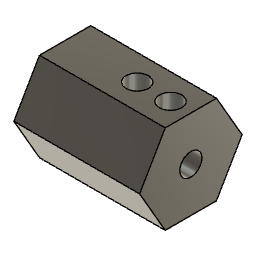
Buggy (Autodesk Fusion 360 archive; units mm, degrees)
design "HexAdapter"
Autodesk Fusion 360 part; units mm, degrees
(part 1 of 3)
sketch "Sketch1" plane through (0, 0, 0) normal (1, 0, 0) x (0, 1, 0)
  line L0 (3.4641, -6) -> (6.9282, 0)
  line L1 (6.9282, 0) -> (3.4641, 6)
  line L2 (3.4641, 6) -> (-3.4641, 6)
  line L3 (-3.4641, 6) -> (-6.9282, 0)
  line L4 (-6.9282, 0) -> (-3.4641, -6)
  line L5 (-3.4641, -6) -> (3.4641, -6)
  dimension "d1" = 6
  measures "d1" distance of origin L5
extrude "Extrude1" add sketch "Sketch1" along normal blind 17
sketch "Sketch2" plane through (0, 0, 0) normal (-1, 0, 0) x (0, -1, 0)
  line L0 (-3.4641, -6) -> (3.4641, -6)
  line L1 (3.4641, -6) -> (6.9282, 0)
  line L2 (6.9282, 0) -> (3.4641, 6)
  line L3 (3.4641, 6) -> (-3.4641, 6)
  line L4 (-3.4641, 6) -> (-6.9282, 0)
  line L5 (-6.9282, 0) -> (-3.4641, -6)
  circle A0 centre (0, 0) radius 1.5
  dimension "d4" = 3
  constraint coincident A0.centre origin
  measures "d4" diameter of A0
extrude "Extrude2" cut sketch "Sketch2" against normal blind 31 contours A0
sketch "Sketch3" plane through (0, 0, 6) normal (0, 0, 1) x (-1, 0, 0)
  line L0 (0, -3.4641) -> (0, 3.4641)
  line L1 (0, 3.4641) -> (-17, 3.4641)
  line L2 (-17, 3.4641) -> (-17, -3.4641)
  line L3 (-17, -3.4641) -> (0, -3.4641)
  line L4 (-17, 0) -> (-14.25, 0)
  circle A0 centre (-14.25, 0) radius 1.5
  line L5 (-14.25, 0) -> (-9.75, 0)
  circle A1 centre (-9.75, 0) radius 1.5
  dimension "d7" = 2.75
  dimension "d8" = 3
  dimension "d9" = 4.5
  dimension "d10" = 3
  constraint midpoint L2 L4.start
  constraint perpendicular L2 L4
  constraint coincident L4.end A0.centre
  constraint parallel L4 L5
  constraint coincident L5.end A1.centre
  measures "d7" distance of L4.start L4.end
  measures "d8" diameter of A0
  measures "d9" distance of L4.end L5.end
  measures "d10" diameter of A1
extrude "Extrude3" cut sketch "Sketch3" against normal blind 6 contours L4 A0 L5 | L4 A0 L5 | A1

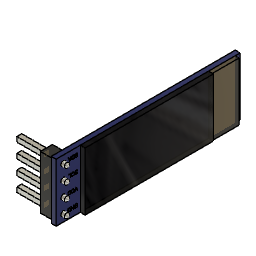
design "OLED mini display"
Autodesk Fusion 360 part; units mm, degrees
sketch "Sketch1" plane through (0, 0, 0) normal (1, 0, 0) x (0, 1, 0)
  line L0 (19, 6) -> (-19, 6)
  line L1 (-19, 6) -> (-19, -6)
  line L2 (-19, -6) -> (19, -6)
  line L3 (19, -6) -> (19, 6)
  line L4 (19, 6) -> (-19, -6) construction
  line L5 (-19, 6) -> (19, -6) construction
  dimension "d1" = 38
  dimension "d2" = 12
  constraint horizontal L0
  constraint perpendicular L0 L1
  constraint parallel L0 L2
  constraint parallel L1 L3
  constraint coincident L4 origin
  constraint coincident L5 origin
  measures "d1" distance of L1.end L2.end
  measures "d2" distance of L0.end L1.end
extrude "Extrude1" add sketch "Sketch1" along normal blind 1 makes body 1
sketch "Sketch2" plane through (1, 0, 0) normal (1, 0, 0) x (0, 1, 0)
  line L0 (19, -6) -> (19, 6)
  line L1 (19, 6) -> (-19, 6)
  line L2 (-19, 6) -> (-19, -6)
  line L3 (-19, -6) -> (19, -6)
  line L4 (-19, 6) -> (-14, 6)
  line L5 (-14, 6) -> (-14, -6)
  line L6 (-14, -6) -> (-19, -6)
  line L7 (-19, -6) -> (-19, 6)
  line L8 (-19, 6) -> (-18, 6)
  line L9 (-18, 6) -> (-18, -6)
  line L10 (-18, 4.5) -> (-18, -4.5)
  circle A0 centre (-17.5, 4.5) radius 0.5
  circle A1 centre (-17.5, 1.5) radius 0.5
  circle A2 centre (-17.5, -1.5) radius 0.5
  circle A3 centre (-17.5, -4.5) radius 0.5
  line L11 (19, 6) -> (18, 6)
  line L12 (18, 6) -> (18, -6)
  line L13 (18, -6) -> (19, -6)
  line L14 (19, -6) -> (19, 6)
  line L15 (18, -6) -> (12.5, -6)
  line L16 (12.5, -6) -> (12.5, 6)
  line L17 (18, 6) -> (12.5, 6)
  line L18 (-14, 6) -> (12.5, 6)
  line L19 (12.5, -6) -> (-14, -6)
  dimension "d5" = 5
  dimension "d6" = 1
  dimension "d7" = 9
  dimension "d8" = 1
  dimension "d11" = 0
  dimension "d12" = -9
  dimension "d13" = 1
  dimension "d14" = 5.5
  constraint coincident L1.end L2.start
  constraint perpendicular L2 L4
  constraint coincident L3 L5.end
  constraint perpendicular L3 L5
  constraint coincident L2.end L3.start
  constraint perpendicular L7 L8
  constraint coincident L6 L9.end
  constraint perpendicular L3 L10
  constraint midpoint L9 L10
  constraint coincident L10.start A0
  constraint coincident L0.end L1.start
  constraint perpendicular L0 L11
  constraint coincident L3 L12.end
  constraint perpendicular L3 L12
  constraint coincident L0.start L3.end
  constraint perpendicular L12 L15
  constraint coincident L1 L16.end
  constraint perpendicular L1 L16
  measures "d5" distance of L1.end L4.end
  measures "d6" distance of L1.end L8.end
  measures "d7" distance of L10.start L10.end
  measures "d8" diameter of A0
  measures "d13" distance of L0.end L11.end
  measures "d14" distance of L12.end L15.end
extrude "Extrude2" add sketch "Sketch2" along normal blind 1 separate body contours L1 L3 L5 L16 L18 L19 makes body 2
extrude "Extrude3" add sketch "Sketch2" along normal blind 0.8 separate body contours L1 L3 L12 L15 L16 L17 makes body 3
extrude "Extrude4" add sketch "Sketch2" along normal blind 1.2 contours A0 | A1 | A2 | A3 bodies 1
chamfer "Chamfer1" distance 0.5 angle 45 4 faces at (2.2, -17.7632, 4.6455) (2.2, -17.7632, 1.6455) (2.2, -17.7632, -1.3545) (2.2, -17.3907, -4.6662) on bodies 1
sketch "Sketch3" plane through (0, 0, 0) normal (-1, 0, 0) x (0, -1, 0)
  line L0 (-19, 6) -> (-19, -6)
  line L1 (-19, -6) -> (19, -6)
  line L2 (19, -6) -> (19, 6)
  line L3 (19, 6) -> (-19, 6)
  line L4 (17, -5) -> (18, -5)
  line L5 (18, -5) -> (18, -4)
  line L6 (18, -4) -> (17, -4)
  line L7 (17, -4) -> (17, -5)
  line L8 (17, -5) -> (18, -4) construction
  line L9 (18, -5) -> (17, -4) construction
  line L10 (17, -2) -> (18, -2)
  line L11 (18, -2) -> (18, -1)
  line L12 (18, -1) -> (17, -1)
  line L13 (17, -1) -> (17, -2)
  line L14 (17, -2) -> (18, -1) construction
  line L15 (18, -2) -> (17, -1) construction
  line L16 (17, 1) -> (18, 1)
  line L17 (18, 1) -> (18, 2)
  line L18 (18, 2) -> (17, 2)
  line L19 (17, 2) -> (17, 1)
  line L20 (17, 1) -> (18, 2) construction
  line L21 (18, 1) -> (17, 2) construction
  line L22 (17, 4) -> (18, 4)
  line L23 (18, 4) -> (18, 5)
  line L24 (18, 5) -> (17, 5)
  line L25 (17, 5) -> (17, 4)
  line L26 (17, 4) -> (18, 5) construction
  line L27 (18, 4) -> (17, 5) construction
  point P0 (17.5, -4.5)
  point P1 (17.5, -1.5)
  point P2 (17.5, 1.5)
  point P3 (17.5, 4.5)
  constraint horizontal L4
  constraint perpendicular L4 L5
  constraint parallel L4 L6
  constraint parallel L5 L7
  constraint coincident L8 P0
  constraint coincident L9 P0
  constraint horizontal L10
  constraint perpendicular L10 L11
  constraint parallel L10 L12
  constraint parallel L11 L13
  constraint coincident L14 P1
  constraint coincident L15 P1
  constraint horizontal L16
  constraint perpendicular L16 L17
  constraint parallel L16 L18
  constraint parallel L17 L19
  constraint coincident L20 P2
  constraint coincident L21 P2
  constraint horizontal L22
  constraint perpendicular L22 L23
  constraint parallel L22 L24
  constraint parallel L23 L25
  constraint coincident L26 P3
  constraint coincident L27 P3
extrude "Extrude5" add sketch "Sketch3" along normal blind 8.5 contours L4 L5 L6 L7 | L10 L11 L12 L13 | L16 L17 L18 L19 | L22 L23 L24 L25 bodies 1
chamfer "Chamfer2" distance 0.4 angle 45 4 faces at (-8.5, -17.3333, -4.3333) (-8.5, -17.3333, -1.3333) (-8.5, -17.3333, 1.6667) (-8.5, -17.3333, 4.6667) on bodies 1
sketch "Sketch4" plane through (0, 0, 0) normal (-1, 0, 0) x (0, -1, 0)
  line L0 (17, 5) -> (18, 5)
  line L1 (18, 5) -> (18, 4)
  line L2 (18, 4) -> (17, 4)
  line L3 (17, 4) -> (17, 5)
  line L4 (17, -4) -> (18, -4)
  line L5 (18, -4) -> (18, -5)
  line L6 (18, -5) -> (17, -5)
  line L7 (17, -5) -> (17, -4)
  line L8 (17, 2) -> (18, 2)
  line L9 (18, 2) -> (18, 1)
  line L10 (18, 1) -> (17, 1)
  line L11 (17, 1) -> (17, 2)
  line L12 (17, -1) -> (18, -1)
  line L13 (18, -1) -> (18, -2)
  line L14 (18, -2) -> (17, -2)
  line L15 (17, -2) -> (17, -1)
  line L16 (-19, 6) -> (-19, -6)
  line L17 (-19, -6) -> (19, -6)
  line L18 (19, -6) -> (19, 6)
  line L19 (19, 6) -> (-19, 6)
  line L20 (19, -5.5) -> (19, 5.5)
  line L21 (19, -5.5) -> (18.75, -5.5)
  line L22 (18.75, -5.5) -> (16.25, -5.5)
  line L23 (18.75, -5.5) -> (18.75, 5.5)
  line L24 (18.75, 5.5) -> (16.25, 5.5)
  line L25 (16.25, 5.5) -> (16.25, -5.5)
  dimension "d25" = 11
  dimension "d27" = 11
  constraint vertical L20
  constraint midpoint L18 L20
  constraint perpendicular L20 L21
  constraint perpendicular L21 L23
  constraint perpendicular L23 L24
  constraint perpendicular L22 L25
  measures "d25" distance of L20.start L20.end
  measures "d27" distance of L21.end L23.end
extrude "Extrude6" add sketch "Sketch4" along normal blind 2.5 contours L22 L23 L24 L25 bodies 1
sketch "Sketch5" plane through (1, 0, 0) normal (1, 0, 0) x (0, 1, 0)
  circle A0 centre (-17.5, -4.5) radius 0.5
  circle A1 centre (-17.5, 4.5) radius 0.5
  circle A2 centre (-17.5, -1.5) radius 0.5
  circle A3 centre (-17.5, 1.5) radius 0.5
  line L0 (19, -6) -> (19, 6)
  line L1 (19, 6) -> (-19, 6)
  line L2 (-19, 6) -> (-19, -6)
  line L3 (-19, -6) -> (19, -6)
  line L4 (-14.5293, -4) -> (-16.5, -4) construction
  line L5 (-16.5, -4) -> (-16.5, -4.767) construction
  line L6 (-16.5, -4.767) -> (-14.5293, -4.767) construction
  line L7 (-14.5293, -4.767) -> (-14.5293, -4) construction
  line L8 (-14.5293, -1) -> (-16.5, -1) construction
  line L9 (-16.5, -1) -> (-16.5, -1.767) construction
  line L10 (-16.5, -1.767) -> (-14.5293, -1.767) construction
  line L11 (-14.5293, -1.767) -> (-14.5293, -1) construction
  line L12 (-14.5293, 2) -> (-16.5, 2) construction
  line L13 (-16.5, 2) -> (-16.5, 1.233) construction
  line L14 (-16.5, 1.233) -> (-14.5293, 1.233) construction
  line L15 (-14.5293, 1.233) -> (-14.5293, 2) construction
  line L16 (-14.5293, 5) -> (-16.5, 5) construction
  line L17 (-16.5, 5) -> (-16.5, 4.233) construction
  line L18 (-16.5, 4.233) -> (-14.5293, 4.233) construction
  line L19 (-14.5293, 4.233) -> (-14.5293, 5) construction
  dimension "d30" = 0.7
  dimension "d31" = 0.7
  dimension "d32" = 0.7
  dimension "d33" = 0.7
  text T0 "GND" font "Arial" height 0.7 align left top in box 1.9707 x 0.767 at (-14.5293, -4) x (-1, 0) y (0, -1) spacing 1 kerned
  text T1 "VCC" font "Arial" height 0.7 align left top in box 1.9707 x 0.767 at (-14.5293, -1) x (-1, 0) y (0, -1) spacing 1 kerned
  text T2 "SCL" font "Arial" height 0.7 align left top in box 1.9707 x 0.767 at (-14.5293, 2) x (-1, 0) y (0, -1) spacing 1 kerned
  text T3 "SDA" font "Arial" height 0.7 align left top in box 1.9707 x 0.767 at (-14.5293, 5) x (-1, 0) y (0, -1) spacing 1 kerned
extrude "Extrude7" cut sketch "Sketch5" against normal blind 0.5 text T0 T1 T2 T3 bodies 1

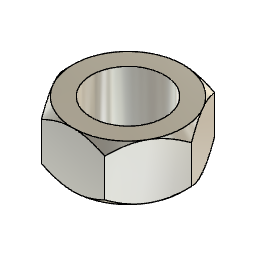
design "2mm Nut"
Autodesk Fusion 360 part; units mm, degrees
sketch "Sketch1" plane through (0, 0, 0) normal (0, 0, 1) x (1, 0, 0)
  circle A0 centre (0, 0) radius 1
  line L0 (-0.866, 1.5) -> (-1.7321, 0)
  line L1 (-1.7321, 0) -> (-0.866, -1.5)
  line L2 (-0.866, -1.5) -> (0.866, -1.5)
  line L3 (0.866, -1.5) -> (1.7321, 0)
  line L4 (1.7321, 0) -> (0.866, 1.5)
  line L5 (0.866, 1.5) -> (-0.866, 1.5)
  dimension "d1" = 2
  constraint coincident A0.centre origin
  measures "d1" diameter of A0
extrude "Extrude1" add sketch "Sketch1" along normal blind 1.5
sketch "Sketch2" plane through (0, 0, 1.5) normal (0, 0, 1) x (-1, 0, 0)
  circle A0 centre (0, 0) radius 1
  line L0 (-0.866, -1.5) -> (0.866, -1.5)
  line L1 (0.866, -1.5) -> (1.7321, 0)
  line L2 (1.7321, 0) -> (0.866, 1.5)
  line L3 (0.866, 1.5) -> (-0.866, 1.5)
  line L4 (-0.866, 1.5) -> (-1.7321, 0)
  line L5 (-1.7321, 0) -> (-0.866, -1.5)
  circle A1 centre (0, 0) radius 1.5
  constraint coincident A0.centre A1.centre
  constraint tangent L0 A1
extrude "Extrude2" cut sketch "Sketch2" against normal blind 3 draft 45 contours A1 keep common part
sketch "Sketch3" plane through (0, 0, 0) normal (0, 0, -1) x (1, 0, 0)
  circle A0 centre (0, 0) radius 1
  line L0 (-0.866, -1.5) -> (0.866, -1.5)
  line L1 (0.866, -1.5) -> (1.7321, 0)
  line L2 (1.7321, 0) -> (0.866, 1.5)
  line L3 (0.866, 1.5) -> (-0.866, 1.5)
  line L4 (-0.866, 1.5) -> (-1.7321, 0)
  line L5 (-1.7321, 0) -> (-0.866, -1.5)
  circle A1 centre (0, 0) radius 1.5
  constraint concentric A0 A1
  constraint tangent L3 A1
extrude "Extrude3" cut sketch "Sketch3" against normal blind 4.4 draft 45 contours A1 keep common part

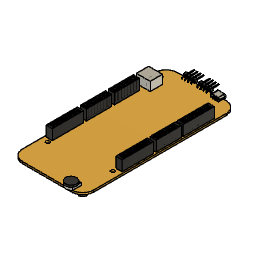
design "S32k144"
Autodesk Fusion 360 part; units mm, degrees
sketch "Sketch1" plane through (0, 0, 0) normal (0, 0, 1) x (1, 0, 0)
  line L0 (0, 0) -> (20, 0)
  line L1 (0, 0) -> (-20, 0)
  line L2 (0, 0) -> (0, 126)
  line L3 (-29, 9) -> (-29, 117)
  line L4 (-20, 126) -> (20, 126)
  line L5 (29, 117) -> (29, 9)
  arc A0 (-20, 126) -> (-29, 117) centre (-20, 117) ccw
  arc A1 (29, 117) -> (20, 126) centre (20, 117) ccw
  arc A2 (20, 0) -> (29, 9) centre (20, 9) ccw
  arc A3 (-29, 9) -> (-20, 0) centre (-20, 9) ccw
  line L6 (-29, 117) -> (-29, 116)
  line L7 (-29, 116) -> (-23.5, 116) construction
  line L8 (-23.5, 116) -> (-23.5, 125.2916) construction
  circle A4 centre (-23.5, 116) radius 1.5
  line L9 (-23.5, 116) -> (-23.5, 24) construction
  circle A5 centre (-23.5, 24) radius 1.5
  line L10 (29, 0) -> (29, 30) construction
  line L11 (29, 30) -> (23.5, 30) construction
  circle A6 centre (23.5, 30) radius 1.5
  line L12 (23.5, 30) -> (23.5, 110) construction
  circle A7 centre (23.5, 110) radius 1.5
  line L13 (29, 108.5) -> (27.7, 108.5) construction
  line L14 (27.7, 108.5) -> (22.7, 108.5)
  line L15 (22.7, 108.5) -> (22.7, 83)
  line L16 (27.7, 108.5) -> (27.7, 83)
  line L17 (22.7, 83) -> (27.7, 83)
  line L18 (25.2, 83) -> (25.2, 81.7) construction
  line L19 (22.7, 81.7) -> (27.7, 81.7)
  line L20 (27.7, 81.7) -> (27.7, 61.2)
  line L21 (22.7, 81.7) -> (22.7, 61.2)
  line L22 (22.7, 61.2) -> (27.7, 61.2)
  line L23 (25.2, 61.2) -> (25.2, 58.9) construction
  line L24 (22.7, 58.9) -> (27.7, 58.9)
  line L25 (27.7, 58.9) -> (27.7, 33.4)
  line L26 (22.7, 58.9) -> (22.7, 33.4)
  line L27 (22.7, 33.4) -> (27.7, 33.4)
  line L28 (-23.5, 116) -> (-23.5, 98) construction
  line L29 (-29, 98) -> (-27.7, 98) construction
  line L30 (-27.7, 98) -> (-22.7, 98)
  line L31 (-27.7, 98) -> (-27.7, 77.5)
  line L32 (-27.7, 77.5) -> (-22.7, 77.5)
  line L33 (-22.7, 98) -> (-22.7, 77.5)
  line L34 (-25.2, 77.5) -> (-25.2, 75.2) construction
  line L35 (-27.7, 75.2) -> (-22.7, 75.2)
  line L36 (-22.7, 75.2) -> (-22.7, 54.7)
  line L37 (-27.7, 75.2) -> (-27.7, 54.7)
  line L38 (-27.7, 54.7) -> (-22.7, 54.7)
  line L39 (-25.2, 54.7) -> (-25.2, 52.4) construction
  line L40 (-27.7, 52.4) -> (-22.7, 52.4)
  line L41 (-27.7, 52.4) -> (-27.7, 26.9)
  line L42 (-22.7, 52.4) -> (-22.7, 26.9)
  line L43 (-27.7, 26.9) -> (-22.7, 26.9)
  line L44 (-25.2, 98) -> (-25.2, 101.5) construction
  line L45 (-29, 101.5) -> (-29, 111.5)
  line L46 (-29, 111.5) -> (-17.5, 111.5)
  line L47 (-17.5, 111.5) -> (-17.5, 101.5)
  line L48 (-17.5, 101.5) -> (-29, 101.5)
  line L49 (-29, 111.5) -> (-28.75, 111.5)
  line L50 (-28.75, 111.5) -> (-28.75, 101.5)
  point P0 (29, 0)
  point P1 (-29, 0)
  point P2 (-29, 126)
  point P3 (29, 126)
  dimension "d1" = 29
  dimension "d2" = 29
  dimension "d3" = 126
  dimension "d4" = 126
  dimension "d5" = 58
  dimension "d6" = 9
  dimension "d7" = 9
  dimension "d8" = 9
  dimension "d9" = 9
  dimension "d13" = 1
  dimension "d15" = 5.5
  dimension "d16" = 9.2916
  dimension "d17" = 3
  dimension "d18" = 92
  dimension "d19" = 3
  dimension "d20" = 30
  dimension "d21" = 5.5
  dimension "d22" = 3
  dimension "d23" = 80
  dimension "d24" = 3
  dimension "d26" = 1.3
  dimension "d27" = 5
  dimension "d29" = 25.5
  dimension "d30" = 1.3
  dimension "d31" = 5
  dimension "d32" = 20.5
  dimension "d34" = 2.3
  dimension "d35" = 5
  dimension "d36" = 25.5
  dimension "d38" = 18
  dimension "d39" = 1.3
  dimension "d40" = 5
  dimension "d41" = 20.5
  dimension "d42" = 5
  dimension "d43" = 2.3
  dimension "d44" = 5
  dimension "d46" = 20.5
  dimension "d47" = 2.3
  dimension "d48" = 5
  dimension "d49" = 25.5
  dimension "d51" = 3.5
  dimension "d52" = 10
  dimension "d53" = 11.5
  dimension "d54" = 10
  dimension "d61" = 0.25
  constraint coincident L0.start L1.start
  constraint horizontal L0
  constraint parallel L0 L1
  constraint perpendicular L0 L2
  constraint perpendicular L1 L3
  constraint perpendicular L2 L4
  constraint coincident P2 L3
  constraint coincident P2 L4
  constraint tangent L3 A0
  constraint tangent L4 A0
  constraint coincident P3 L4
  constraint coincident P3 L5
  constraint tangent L4 A1
  constraint tangent L5 A1
  constraint coincident P0 L0
  constraint coincident P0 L5
  constraint tangent L0 A2
  constraint tangent L5 A2
  constraint coincident P1 L1
  constraint coincident P1 L3
  constraint tangent L1 A3
  constraint tangent L3 A3
  constraint parallel L3 L6
  constraint coincident A0 L8.end
  constraint perpendicular L7 L8
  constraint coincident L7.end L8.start
  constraint perpendicular L7 L9
  constraint coincident L9.end A5.centre
  constraint coincident P0 L10.start
  constraint parallel L5 L10
  constraint perpendicular L5 L11
  constraint coincident L11.end A6.centre
  constraint perpendicular L11 L12
  constraint coincident L12.end A7.centre
  constraint coincident L5 L13.start
  constraint perpendicular L5 L13
  constraint parallel L13 L14
  constraint perpendicular L14 L15
  constraint perpendicular L14 L16
  constraint midpoint L17 L18.start
  constraint perpendicular L17 L18
  constraint perpendicular L18 L19
  constraint perpendicular L19 L20
  constraint perpendicular L19 L21
  constraint tangent A7 L14
  constraint midpoint L22 L23.start
  constraint perpendicular L22 L23
  constraint perpendicular L12 L24
  constraint perpendicular L24 L25
  constraint perpendicular L24 L26
  constraint perpendicular L7 L28
  constraint coincident L3 L29.start
  constraint perpendicular L3 L29
  constraint parallel L29 L30
  constraint perpendicular L30 L31
  constraint perpendicular L31 L32
  constraint midpoint L32 L34.start
  constraint perpendicular L32 L34
  constraint perpendicular L9 L35
  constraint perpendicular L35 L36
  constraint perpendicular L35 L37
  constraint midpoint L38 L39.start
  constraint perpendicular L38 L39
  constraint perpendicular L39 L40
  constraint perpendicular L40 L41
  constraint perpendicular L40 L42
  constraint midpoint L30 L44.start
  constraint perpendicular L30 L44
  constraint coincident L3 L45.start
  constraint parallel L3 L45
  constraint perpendicular L45 L46
  constraint perpendicular L46 L47
  constraint perpendicular L45 L49
  constraint coincident L48 L50.end
  constraint perpendicular L48 L50
  measures "d1" distance of L0.start P0
  measures "d2" distance of L0.start P1
  measures "d3" distance of L0.start L2.end
  measures "d4" distance of P1 P2
  measures "d5" distance of P2 P3
  measures "d6" radius of A0
  measures "d7" radius of A1
  measures "d8" radius of A2
  measures "d9" radius of A3
  measures "d13" distance of L3.end L6.end
  measures "d15" distance of L6.end L7.end
  measures "d16" distance of L7.end L8.end
  measures "d17" diameter of A4
  measures "d18" distance of L7.end L9.end
  measures "d19" diameter of A5
  measures "d20" distance of P0 L10.end
  measures "d21" distance of L10.end L11.end
  measures "d22" diameter of A6
  measures "d23" distance of L11.end L12.end
  measures "d24" diameter of A7
  measures "d26" distance of L13.start L13.end
  measures "d27" distance of L13.end L14.end
  measures "d29" distance of L13.end L16.end
  measures "d30" distance of L18.start L18.end
  measures "d31" distance of L19.start L19.end
  measures "d32" distance of L19.end L20.end
  measures "d34" distance of L23.start L23.end
  measures "d35" distance of L24.start L24.end
  measures "d36" distance of L24.end L25.end
  measures "d38" distance of L7.end L28.end
  measures "d39" distance of L29.start L29.end
  measures "d40" distance of L29.end L30.end
  measures "d41" distance of L29.end L31.end
  measures "d42" distance of L31.end L32.end
  measures "d43" distance of L34.start L34.end
  measures "d44" distance of L35.start L35.end
  measures "d46" distance of L35.start L37.end
  measures "d47" distance of L39.start L39.end
  measures "d48" distance of L40.start L40.end
  measures "d49" distance of L40.start L41.end
  measures "d51" distance of L44.start L44.end
  measures "d52" distance of L45.start L45.end
  measures "d53" distance of L45.end L46.end
  measures "d54" distance of L46.end L47.end
  measures "d61" distance of L45.end L49.end
extrude "Extrude1" add sketch "Sketch1" along normal blind 1.5 contours L0 L2 L4 L5 A1 A2 | L1 L2 L3 L4 A0 A3 L6 L46 L47 L48 L49 | L3 L45 L46 L48 L49 L50 | L46 L47 L48 L50 | A4 | A5 | A6 | A7 | L14 L15 L16 L17 | L19 L20 L21 L22 | L24 L25 L26 L27 | L30 L31 L32 L33 | L35 L36 L37 L38 | L40 L41 L42 L43 makes body 1
extrude "Extrude2" cut sketch "Sketch1" along normal blind 33 contours A4 | A5 | A6 | A7 bodies 1
extrude "Extrude3" add sketch "Sketch1" along normal blind 10 contours L14 L15 L16 L17 | L19 L20 L21 L22 | L24 L25 L26 L27 | L30 L31 L32 L33 | L35 L36 L37 L38 | L40 L41 L42 L43 bodies 1
extrude "Extrude4" add sketch "Sketch1" along normal blind 8.7 contours L46 L47 L48 L50 bodies 1
sketch "Sketch2" plane through (-28.75, 0, 0) normal (-1, 0, 0) x (0, -1, 0)
  line L0 (-111.5, 1.5) -> (-101.5, 1.5)
  line L1 (-101.5, 1.5) -> (-101.5, 8.7)
  line L2 (-101.5, 8.7) -> (-111.5, 8.7)
  line L3 (-111.5, 8.7) -> (-111.5, 1.5)
  circle A0 centre (-105, 5) radius 3
  dimension "d64" = 6
  measures "d64" diameter of A0
extrude "Extrude5" cut sketch "Sketch2" against normal blind 8 contours A0 bodies 1
sketch "Sketch3" plane through (-20.75, 0, 0) normal (-1, 0, 0) x (0, -1, 0)
  circle A0 centre (-105, 5) radius 3
  circle A1 centre (-105, 5) radius 1
  dimension "d67" = 2
  constraint concentric A0 A1
  measures "d67" diameter of A1
extrude "Extrude6" add sketch "Sketch3" along normal blind 7 contours A1 bodies 1
fillet "Fillet1" radius 1 1 faces at (-27.75, 105.0787, 4.4037) on bodies 1
sketch "Sketch4" plane through (0, 0, 10) normal (0, 0, 1) x (-1, 0, 0)
  line L0 (27.7, -98) -> (27.7, -77.5)
  line L1 (27.7, -77.5) -> (22.7, -77.5)
  line L2 (22.7, -77.5) -> (22.7, -98)
  line L3 (22.7, -98) -> (27.7, -98)
  line L4 (27, -97) -> (25.5, -97)
  line L5 (25.5, -97) -> (25.5, -95.5)
  line L6 (25.5, -95.5) -> (27, -95.5)
  line L7 (27, -95.5) -> (27, -97)
  line L8 (24.7, -97) -> (23.2, -97)
  line L9 (24.7, -95.5) -> (24.7, -97)
  line L10 (23.2, -95.5) -> (24.7, -95.5)
  line L11 (23.2, -97) -> (23.2, -95.5)
  line L12 (27, -94.5714) -> (25.5, -94.5714)
  line L13 (27, -93.0714) -> (27, -94.5714)
  line L14 (25.5, -93.0714) -> (27, -93.0714)
  line L15 (25.5, -94.5714) -> (25.5, -93.0714)
  line L16 (24.7, -94.5714) -> (23.2, -94.5714)
  line L17 (24.7, -93.0714) -> (24.7, -94.5714)
  line L18 (23.2, -93.0714) -> (24.7, -93.0714)
  line L19 (23.2, -94.5714) -> (23.2, -93.0714)
  line L20 (27, -92.1429) -> (25.5, -92.1429)
  line L21 (27, -90.6429) -> (27, -92.1429)
  line L22 (25.5, -90.6429) -> (27, -90.6429)
  line L23 (25.5, -92.1429) -> (25.5, -90.6429)
  line L24 (24.7, -92.1429) -> (23.2, -92.1429)
  line L25 (24.7, -90.6429) -> (24.7, -92.1429)
  line L26 (23.2, -90.6429) -> (24.7, -90.6429)
  line L27 (23.2, -92.1429) -> (23.2, -90.6429)
  line L28 (27, -89.7143) -> (25.5, -89.7143)
  line L29 (27, -88.2143) -> (27, -89.7143)
  line L30 (25.5, -88.2143) -> (27, -88.2143)
  line L31 (25.5, -89.7143) -> (25.5, -88.2143)
  line L32 (24.7, -89.7143) -> (23.2, -89.7143)
  line L33 (24.7, -88.2143) -> (24.7, -89.7143)
  line L34 (23.2, -88.2143) -> (24.7, -88.2143)
  line L35 (23.2, -89.7143) -> (23.2, -88.2143)
  line L36 (27, -87.2857) -> (25.5, -87.2857)
  line L37 (27, -85.7857) -> (27, -87.2857)
  line L38 (25.5, -85.7857) -> (27, -85.7857)
  line L39 (25.5, -87.2857) -> (25.5, -85.7857)
  line L40 (24.7, -87.2857) -> (23.2, -87.2857)
  line L41 (24.7, -85.7857) -> (24.7, -87.2857)
  line L42 (23.2, -85.7857) -> (24.7, -85.7857)
  line L43 (23.2, -87.2857) -> (23.2, -85.7857)
  line L44 (27, -84.8571) -> (25.5, -84.8571)
  line L45 (27, -83.3571) -> (27, -84.8571)
  line L46 (25.5, -83.3571) -> (27, -83.3571)
  line L47 (25.5, -84.8571) -> (25.5, -83.3571)
  line L48 (24.7, -84.8571) -> (23.2, -84.8571)
  line L49 (24.7, -83.3571) -> (24.7, -84.8571)
  line L50 (23.2, -83.3571) -> (24.7, -83.3571)
  line L51 (23.2, -84.8571) -> (23.2, -83.3571)
  line L52 (27, -82.4286) -> (25.5, -82.4286)
  line L53 (27, -80.9286) -> (27, -82.4286)
  line L54 (25.5, -80.9286) -> (27, -80.9286)
  line L55 (25.5, -82.4286) -> (25.5, -80.9286)
  line L56 (24.7, -82.4286) -> (23.2, -82.4286)
  line L57 (24.7, -80.9286) -> (24.7, -82.4286)
  line L58 (23.2, -80.9286) -> (24.7, -80.9286)
  line L59 (23.2, -82.4286) -> (23.2, -80.9286)
  line L60 (27, -80) -> (25.5, -80)
  line L61 (27, -78.5) -> (27, -80)
  line L62 (25.5, -78.5) -> (27, -78.5)
  line L63 (25.5, -80) -> (25.5, -78.5)
  line L64 (24.7, -80) -> (23.2, -80)
  line L65 (24.7, -78.5) -> (24.7, -80)
  line L66 (23.2, -78.5) -> (24.7, -78.5)
  line L67 (23.2, -80) -> (23.2, -78.5)
  line L68 (27, -74) -> (25.5, -74)
  line L69 (27, -72.5) -> (27, -74)
  line L70 (25.5, -72.5) -> (27, -72.5)
  line L71 (25.5, -74) -> (25.5, -72.5)
  line L72 (27, -51) -> (25.5, -51)
  line L73 (27, -49.5) -> (27, -51)
  line L74 (25.5, -49.5) -> (27, -49.5)
  line L75 (25.5, -51) -> (25.5, -49.5)
  line L76 (-23.5, -56) -> (-23.5, -57.5)
  line L77 (-25, -57.5) -> (-25, -56)
  line L78 (-25, -56) -> (-23.5, -56)
  line L79 (-23.5, -57.5) -> (-25, -57.5)
  line L80 (-23.5, -78.5) -> (-23.5, -80)
  line L81 (-25, -80) -> (-25, -78.5)
  line L82 (-25, -78.5) -> (-23.5, -78.5)
  line L83 (-23.5, -80) -> (-25, -80)
  line L84 (-25, -107) -> (-25, -105.5)
  line L85 (-23.5, -105.5) -> (-23.5, -107)
  line L86 (-23.5, -107) -> (-25, -107)
  line L87 (-25, -105.5) -> (-23.5, -105.5)
  line L88 (24.7, -74) -> (23.2, -74)
  line L89 (24.7, -72.5) -> (24.7, -74)
  line L90 (23.2, -74) -> (23.2, -72.5)
  line L91 (23.2, -72.5) -> (24.7, -72.5)
  line L92 (27, -71.5714) -> (25.5, -71.5714)
  line L93 (27, -70.0714) -> (27, -71.5714)
  line L94 (25.5, -71.5714) -> (25.5, -70.0714)
  line L95 (25.5, -70.0714) -> (27, -70.0714)
  line L96 (24.7, -71.5714) -> (23.2, -71.5714)
  line L97 (24.7, -70.0714) -> (24.7, -71.5714)
  line L98 (23.2, -71.5714) -> (23.2, -70.0714)
  line L99 (23.2, -70.0714) -> (24.7, -70.0714)
  line L100 (27, -69.1429) -> (25.5, -69.1429)
  line L101 (27, -67.6429) -> (27, -69.1429)
  line L102 (25.5, -69.1429) -> (25.5, -67.6429)
  line L103 (25.5, -67.6429) -> (27, -67.6429)
  line L104 (24.7, -69.1429) -> (23.2, -69.1429)
  line L105 (24.7, -67.6429) -> (24.7, -69.1429)
  line L106 (23.2, -69.1429) -> (23.2, -67.6429)
  line L107 (23.2, -67.6429) -> (24.7, -67.6429)
  line L108 (27, -66.7143) -> (25.5, -66.7143)
  line L109 (27, -65.2143) -> (27, -66.7143)
  line L110 (25.5, -66.7143) -> (25.5, -65.2143)
  line L111 (25.5, -65.2143) -> (27, -65.2143)
  line L112 (24.7, -66.7143) -> (23.2, -66.7143)
  line L113 (24.7, -65.2143) -> (24.7, -66.7143)
  line L114 (23.2, -66.7143) -> (23.2, -65.2143)
  line L115 (23.2, -65.2143) -> (24.7, -65.2143)
  line L116 (27, -64.2857) -> (25.5, -64.2857)
  line L117 (27, -62.7857) -> (27, -64.2857)
  line L118 (25.5, -64.2857) -> (25.5, -62.7857)
  line L119 (25.5, -62.7857) -> (27, -62.7857)
  line L120 (24.7, -64.2857) -> (23.2, -64.2857)
  line L121 (24.7, -62.7857) -> (24.7, -64.2857)
  line L122 (23.2, -64.2857) -> (23.2, -62.7857)
  line L123 (23.2, -62.7857) -> (24.7, -62.7857)
  line L124 (27, -61.8571) -> (25.5, -61.8571)
  line L125 (27, -60.3571) -> (27, -61.8571)
  line L126 (25.5, -61.8571) -> (25.5, -60.3571)
  line L127 (25.5, -60.3571) -> (27, -60.3571)
  line L128 (24.7, -61.8571) -> (23.2, -61.8571)
  line L129 (24.7, -60.3571) -> (24.7, -61.8571)
  line L130 (23.2, -61.8571) -> (23.2, -60.3571)
  line L131 (23.2, -60.3571) -> (24.7, -60.3571)
  line L132 (27, -59.4286) -> (25.5, -59.4286)
  line L133 (27, -57.9286) -> (27, -59.4286)
  line L134 (25.5, -59.4286) -> (25.5, -57.9286)
  line L135 (25.5, -57.9286) -> (27, -57.9286)
  line L136 (24.7, -59.4286) -> (23.2, -59.4286)
  line L137 (24.7, -57.9286) -> (24.7, -59.4286)
  line L138 (23.2, -59.4286) -> (23.2, -57.9286)
  line L139 (23.2, -57.9286) -> (24.7, -57.9286)
  line L140 (27, -57) -> (25.5, -57)
  line L141 (27, -55.5) -> (27, -57)
  line L142 (25.5, -57) -> (25.5, -55.5)
  line L143 (25.5, -55.5) -> (27, -55.5)
  line L144 (24.7, -57) -> (23.2, -57)
  line L145 (24.7, -55.5) -> (24.7, -57)
  line L146 (23.2, -57) -> (23.2, -55.5)
  line L147 (23.2, -55.5) -> (24.7, -55.5)
  line L148 (25, -51) -> (23.5, -51)
  line L149 (25, -49.5) -> (25, -51)
  line L150 (23.5, -49.5) -> (25, -49.5)
  line L151 (23.5, -51) -> (23.5, -49.5)
  line L152 (27, -48.6667) -> (25.5, -48.6667)
  line L153 (27, -47.1667) -> (27, -48.6667)
  line L154 (25.5, -47.1667) -> (27, -47.1667)
  line L155 (25.5, -48.6667) -> (25.5, -47.1667)
  line L156 (25, -48.6667) -> (23.5, -48.6667)
  line L157 (25, -47.1667) -> (25, -48.6667)
  line L158 (23.5, -47.1667) -> (25, -47.1667)
  line L159 (23.5, -48.6667) -> (23.5, -47.1667)
  line L160 (27, -46.3333) -> (25.5, -46.3333)
  line L161 (27, -44.8333) -> (27, -46.3333)
  line L162 (25.5, -44.8333) -> (27, -44.8333)
  line L163 (25.5, -46.3333) -> (25.5, -44.8333)
  line L164 (25, -46.3333) -> (23.5, -46.3333)
  line L165 (25, -44.8333) -> (25, -46.3333)
  line L166 (23.5, -44.8333) -> (25, -44.8333)
  line L167 (23.5, -46.3333) -> (23.5, -44.8333)
  line L168 (27, -44) -> (25.5, -44)
  line L169 (27, -42.5) -> (27, -44)
  line L170 (25.5, -42.5) -> (27, -42.5)
  line L171 (25.5, -44) -> (25.5, -42.5)
  line L172 (25, -44) -> (23.5, -44)
  line L173 (25, -42.5) -> (25, -44)
  line L174 (23.5, -42.5) -> (25, -42.5)
  line L175 (23.5, -44) -> (23.5, -42.5)
  line L176 (27, -41.6667) -> (25.5, -41.6667)
  line L177 (27, -40.1667) -> (27, -41.6667)
  line L178 (25.5, -40.1667) -> (27, -40.1667)
  line L179 (25.5, -41.6667) -> (25.5, -40.1667)
  line L180 (25, -41.6667) -> (23.5, -41.6667)
  line L181 (25, -40.1667) -> (25, -41.6667)
  line L182 (23.5, -40.1667) -> (25, -40.1667)
  line L183 (23.5, -41.6667) -> (23.5, -40.1667)
  line L184 (27, -39.3333) -> (25.5, -39.3333)
  line L185 (27, -37.8333) -> (27, -39.3333)
  line L186 (25.5, -37.8333) -> (27, -37.8333)
  line L187 (25.5, -39.3333) -> (25.5, -37.8333)
  line L188 (25, -39.3333) -> (23.5, -39.3333)
  line L189 (25, -37.8333) -> (25, -39.3333)
  line L190 (23.5, -37.8333) -> (25, -37.8333)
  line L191 (23.5, -39.3333) -> (23.5, -37.8333)
  line L192 (27, -37) -> (25.5, -37)
  line L193 (27, -35.5) -> (27, -37)
  line L194 (25.5, -35.5) -> (27, -35.5)
  line L195 (25.5, -37) -> (25.5, -35.5)
  line L196 (25, -37) -> (23.5, -37)
  line L197 (25, -35.5) -> (25, -37)
  line L198 (23.5, -35.5) -> (25, -35.5)
  line L199 (23.5, -37) -> (23.5, -35.5)
  line L200 (27, -34.6667) -> (25.5, -34.6667)
  line L201 (27, -33.1667) -> (27, -34.6667)
  line L202 (25.5, -33.1667) -> (27, -33.1667)
  line L203 (25.5, -34.6667) -> (25.5, -33.1667)
  line L204 (25, -34.6667) -> (23.5, -34.6667)
  line L205 (25, -33.1667) -> (25, -34.6667)
  line L206 (23.5, -33.1667) -> (25, -33.1667)
  line L207 (23.5, -34.6667) -> (23.5, -33.1667)
  line L208 (27, -32.3333) -> (25.5, -32.3333)
  line L209 (27, -30.8333) -> (27, -32.3333)
  line L210 (25.5, -30.8333) -> (27, -30.8333)
  line L211 (25.5, -32.3333) -> (25.5, -30.8333)
  line L212 (25, -32.3333) -> (23.5, -32.3333)
  line L213 (25, -30.8333) -> (25, -32.3333)
  line L214 (23.5, -30.8333) -> (25, -30.8333)
  line L215 (23.5, -32.3333) -> (23.5, -30.8333)
  line L216 (27, -30) -> (25.5, -30)
  line L217 (27, -28.5) -> (27, -30)
  line L218 (25.5, -28.5) -> (27, -28.5)
  line L219 (25.5, -30) -> (25.5, -28.5)
  line L220 (25, -30) -> (23.5, -30)
  line L221 (25, -28.5) -> (25, -30)
  line L222 (23.5, -28.5) -> (25, -28.5)
  line L223 (23.5, -30) -> (23.5, -28.5)
  line L224 (-27, -107) -> (-27, -105.5)
  line L225 (-25.5, -105.5) -> (-25.5, -107)
  line L226 (-27, -105.5) -> (-25.5, -105.5)
  line L227 (-25.5, -107) -> (-27, -107)
  line L228 (-25, -104.6667) -> (-25, -103.1667)
  line L229 (-23.5, -103.1667) -> (-23.5, -104.6667)
  line L230 (-25, -103.1667) -> (-23.5, -103.1667)
  line L231 (-23.5, -104.6667) -> (-25, -104.6667)
  line L232 (-27, -104.6667) -> (-27, -103.1667)
  line L233 (-25.5, -103.1667) -> (-25.5, -104.6667)
  line L234 (-27, -103.1667) -> (-25.5, -103.1667)
  line L235 (-25.5, -104.6667) -> (-27, -104.6667)
  line L236 (-25, -102.3333) -> (-25, -100.8333)
  line L237 (-23.5, -100.8333) -> (-23.5, -102.3333)
  line L238 (-25, -100.8333) -> (-23.5, -100.8333)
  line L239 (-23.5, -102.3333) -> (-25, -102.3333)
  line L240 (-27, -102.3333) -> (-27, -100.8333)
  line L241 (-25.5, -100.8333) -> (-25.5, -102.3333)
  line L242 (-27, -100.8333) -> (-25.5, -100.8333)
  line L243 (-25.5, -102.3333) -> (-27, -102.3333)
  line L244 (-25, -100) -> (-25, -98.5)
  line L245 (-23.5, -98.5) -> (-23.5, -100)
  line L246 (-25, -98.5) -> (-23.5, -98.5)
  line L247 (-23.5, -100) -> (-25, -100)
  line L248 (-27, -100) -> (-27, -98.5)
  line L249 (-25.5, -98.5) -> (-25.5, -100)
  line L250 (-27, -98.5) -> (-25.5, -98.5)
  line L251 (-25.5, -100) -> (-27, -100)
  line L252 (-25, -97.6667) -> (-25, -96.1667)
  line L253 (-23.5, -96.1667) -> (-23.5, -97.6667)
  line L254 (-25, -96.1667) -> (-23.5, -96.1667)
  line L255 (-23.5, -97.6667) -> (-25, -97.6667)
  line L256 (-27, -97.6667) -> (-27, -96.1667)
  line L257 (-25.5, -96.1667) -> (-25.5, -97.6667)
  line L258 (-27, -96.1667) -> (-25.5, -96.1667)
  line L259 (-25.5, -97.6667) -> (-27, -97.6667)
  line L260 (-25, -95.3333) -> (-25, -93.8333)
  line L261 (-23.5, -93.8333) -> (-23.5, -95.3333)
  line L262 (-25, -93.8333) -> (-23.5, -93.8333)
  line L263 (-23.5, -95.3333) -> (-25, -95.3333)
  line L264 (-27, -95.3333) -> (-27, -93.8333)
  line L265 (-25.5, -93.8333) -> (-25.5, -95.3333)
  line L266 (-27, -93.8333) -> (-25.5, -93.8333)
  line L267 (-25.5, -95.3333) -> (-27, -95.3333)
  line L268 (-25, -93) -> (-25, -91.5)
  line L269 (-23.5, -91.5) -> (-23.5, -93)
  line L270 (-25, -91.5) -> (-23.5, -91.5)
  line L271 (-23.5, -93) -> (-25, -93)
  line L272 (-27, -93) -> (-27, -91.5)
  line L273 (-25.5, -91.5) -> (-25.5, -93)
  line L274 (-27, -91.5) -> (-25.5, -91.5)
  line L275 (-25.5, -93) -> (-27, -93)
  line L276 (-25, -90.6667) -> (-25, -89.1667)
  line L277 (-23.5, -89.1667) -> (-23.5, -90.6667)
  line L278 (-25, -89.1667) -> (-23.5, -89.1667)
  line L279 (-23.5, -90.6667) -> (-25, -90.6667)
  line L280 (-27, -90.6667) -> (-27, -89.1667)
  line L281 (-25.5, -89.1667) -> (-25.5, -90.6667)
  line L282 (-27, -89.1667) -> (-25.5, -89.1667)
  line L283 (-25.5, -90.6667) -> (-27, -90.6667)
  line L284 (-25, -88.3333) -> (-25, -86.8333)
  line L285 (-23.5, -86.8333) -> (-23.5, -88.3333)
  line L286 (-25, -86.8333) -> (-23.5, -86.8333)
  line L287 (-23.5, -88.3333) -> (-25, -88.3333)
  line L288 (-27, -88.3333) -> (-27, -86.8333)
  line L289 (-25.5, -86.8333) -> (-25.5, -88.3333)
  line L290 (-27, -86.8333) -> (-25.5, -86.8333)
  line L291 (-25.5, -88.3333) -> (-27, -88.3333)
  line L292 (-25, -86) -> (-25, -84.5)
  line L293 (-23.5, -84.5) -> (-23.5, -86)
  line L294 (-25, -84.5) -> (-23.5, -84.5)
  line L295 (-23.5, -86) -> (-25, -86)
  line L296 (-27, -86) -> (-27, -84.5)
  line L297 (-25.5, -84.5) -> (-25.5, -86)
  line L298 (-27, -84.5) -> (-25.5, -84.5)
  line L299 (-25.5, -86) -> (-27, -86)
  line L300 (-27, -78.5) -> (-25.5, -78.5)
  line L301 (-27, -80) -> (-27, -78.5)
  line L302 (-25.5, -78.5) -> (-25.5, -80)
  line L303 (-25.5, -80) -> (-27, -80)
  line L304 (-25, -76.2143) -> (-23.5, -76.2143)
  line L305 (-25, -77.7143) -> (-25, -76.2143)
  line L306 (-23.5, -76.2143) -> (-23.5, -77.7143)
  line L307 (-23.5, -77.7143) -> (-25, -77.7143)
  line L308 (-27, -76.2143) -> (-25.5, -76.2143)
  line L309 (-27, -77.7143) -> (-27, -76.2143)
  line L310 (-25.5, -76.2143) -> (-25.5, -77.7143)
  line L311 (-25.5, -77.7143) -> (-27, -77.7143)
  line L312 (-25, -73.9286) -> (-23.5, -73.9286)
  line L313 (-25, -75.4286) -> (-25, -73.9286)
  line L314 (-23.5, -73.9286) -> (-23.5, -75.4286)
  line L315 (-23.5, -75.4286) -> (-25, -75.4286)
  line L316 (-27, -73.9286) -> (-25.5, -73.9286)
  line L317 (-27, -75.4286) -> (-27, -73.9286)
  line L318 (-25.5, -73.9286) -> (-25.5, -75.4286)
  line L319 (-25.5, -75.4286) -> (-27, -75.4286)
  line L320 (-25, -71.6429) -> (-23.5, -71.6429)
  line L321 (-25, -73.1429) -> (-25, -71.6429)
  line L322 (-23.5, -71.6429) -> (-23.5, -73.1429)
  line L323 (-23.5, -73.1429) -> (-25, -73.1429)
  line L324 (-27, -71.6429) -> (-25.5, -71.6429)
  line L325 (-27, -73.1429) -> (-27, -71.6429)
  line L326 (-25.5, -71.6429) -> (-25.5, -73.1429)
  line L327 (-25.5, -73.1429) -> (-27, -73.1429)
  line L328 (-25, -69.3571) -> (-23.5, -69.3571)
  line L329 (-25, -70.8571) -> (-25, -69.3571)
  line L330 (-23.5, -69.3571) -> (-23.5, -70.8571)
  line L331 (-23.5, -70.8571) -> (-25, -70.8571)
  line L332 (-27, -69.3571) -> (-25.5, -69.3571)
  line L333 (-27, -70.8571) -> (-27, -69.3571)
  line L334 (-25.5, -69.3571) -> (-25.5, -70.8571)
  line L335 (-25.5, -70.8571) -> (-27, -70.8571)
  line L336 (-25, -67.0714) -> (-23.5, -67.0714)
  line L337 (-25, -68.5714) -> (-25, -67.0714)
  line L338 (-23.5, -67.0714) -> (-23.5, -68.5714)
  line L339 (-23.5, -68.5714) -> (-25, -68.5714)
  line L340 (-27, -67.0714) -> (-25.5, -67.0714)
  line L341 (-27, -68.5714) -> (-27, -67.0714)
  line L342 (-25.5, -67.0714) -> (-25.5, -68.5714)
  line L343 (-25.5, -68.5714) -> (-27, -68.5714)
  line L344 (-25, -64.7857) -> (-23.5, -64.7857)
  line L345 (-25, -66.2857) -> (-25, -64.7857)
  line L346 (-23.5, -64.7857) -> (-23.5, -66.2857)
  line L347 (-23.5, -66.2857) -> (-25, -66.2857)
  line L348 (-27, -64.7857) -> (-25.5, -64.7857)
  line L349 (-27, -66.2857) -> (-27, -64.7857)
  line L350 (-25.5, -64.7857) -> (-25.5, -66.2857)
  line L351 (-25.5, -66.2857) -> (-27, -66.2857)
  line L352 (-25, -62.5) -> (-23.5, -62.5)
  line L353 (-25, -64) -> (-25, -62.5)
  line L354 (-23.5, -62.5) -> (-23.5, -64)
  line L355 (-23.5, -64) -> (-25, -64)
  line L356 (-27, -62.5) -> (-25.5, -62.5)
  line L357 (-27, -64) -> (-27, -62.5)
  line L358 (-25.5, -62.5) -> (-25.5, -64)
  line L359 (-25.5, -64) -> (-27, -64)
  line L360 (-27, -56) -> (-25.5, -56)
  line L361 (-25.5, -56) -> (-25.5, -57.5)
  line L362 (-25.5, -57.5) -> (-27, -57.5)
  line L363 (-27, -57.5) -> (-27, -56)
  line L364 (-25, -53.6667) -> (-23.5, -53.6667)
  line L365 (-23.5, -53.6667) -> (-23.5, -55.1667)
  line L366 (-23.5, -55.1667) -> (-25, -55.1667)
  line L367 (-25, -55.1667) -> (-25, -53.6667)
  line L368 (-27, -53.6667) -> (-25.5, -53.6667)
  line L369 (-25.5, -53.6667) -> (-25.5, -55.1667)
  line L370 (-25.5, -55.1667) -> (-27, -55.1667)
  line L371 (-27, -55.1667) -> (-27, -53.6667)
  line L372 (-25, -51.3333) -> (-23.5, -51.3333)
  line L373 (-23.5, -51.3333) -> (-23.5, -52.8333)
  line L374 (-23.5, -52.8333) -> (-25, -52.8333)
  line L375 (-25, -52.8333) -> (-25, -51.3333)
  line L376 (-27, -51.3333) -> (-25.5, -51.3333)
  line L377 (-25.5, -51.3333) -> (-25.5, -52.8333)
  line L378 (-25.5, -52.8333) -> (-27, -52.8333)
  line L379 (-27, -52.8333) -> (-27, -51.3333)
  line L380 (-25, -49) -> (-23.5, -49)
  line L381 (-23.5, -49) -> (-23.5, -50.5)
  line L382 (-23.5, -50.5) -> (-25, -50.5)
  line L383 (-25, -50.5) -> (-25, -49)
  line L384 (-27, -49) -> (-25.5, -49)
  line L385 (-25.5, -49) -> (-25.5, -50.5)
  line L386 (-25.5, -50.5) -> (-27, -50.5)
  line L387 (-27, -50.5) -> (-27, -49)
  line L388 (-25, -46.6667) -> (-23.5, -46.6667)
  line L389 (-23.5, -46.6667) -> (-23.5, -48.1667)
  line L390 (-23.5, -48.1667) -> (-25, -48.1667)
  line L391 (-25, -48.1667) -> (-25, -46.6667)
  line L392 (-27, -46.6667) -> (-25.5, -46.6667)
  line L393 (-25.5, -46.6667) -> (-25.5, -48.1667)
  line L394 (-25.5, -48.1667) -> (-27, -48.1667)
  line L395 (-27, -48.1667) -> (-27, -46.6667)
  line L396 (-25, -44.3333) -> (-23.5, -44.3333)
  line L397 (-23.5, -44.3333) -> (-23.5, -45.8333)
  line L398 (-23.5, -45.8333) -> (-25, -45.8333)
  line L399 (-25, -45.8333) -> (-25, -44.3333)
  line L400 (-27, -44.3333) -> (-25.5, -44.3333)
  line L401 (-25.5, -44.3333) -> (-25.5, -45.8333)
  line L402 (-25.5, -45.8333) -> (-27, -45.8333)
  line L403 (-27, -45.8333) -> (-27, -44.3333)
  line L404 (-25, -42) -> (-23.5, -42)
  line L405 (-23.5, -42) -> (-23.5, -43.5)
  line L406 (-23.5, -43.5) -> (-25, -43.5)
  line L407 (-25, -43.5) -> (-25, -42)
  line L408 (-27, -42) -> (-25.5, -42)
  line L409 (-25.5, -42) -> (-25.5, -43.5)
  line L410 (-25.5, -43.5) -> (-27, -43.5)
  line L411 (-27, -43.5) -> (-27, -42)
  line L412 (-25, -39.6667) -> (-23.5, -39.6667)
  line L413 (-23.5, -39.6667) -> (-23.5, -41.1667)
  line L414 (-23.5, -41.1667) -> (-25, -41.1667)
  line L415 (-25, -41.1667) -> (-25, -39.6667)
  line L416 (-27, -39.6667) -> (-25.5, -39.6667)
  line L417 (-25.5, -39.6667) -> (-25.5, -41.1667)
  line L418 (-25.5, -41.1667) -> (-27, -41.1667)
  line L419 (-27, -41.1667) -> (-27, -39.6667)
  line L420 (-25, -37.3333) -> (-23.5, -37.3333)
  line L421 (-23.5, -37.3333) -> (-23.5, -38.8333)
  line L422 (-23.5, -38.8333) -> (-25, -38.8333)
  line L423 (-25, -38.8333) -> (-25, -37.3333)
  line L424 (-27, -37.3333) -> (-25.5, -37.3333)
  line L425 (-25.5, -37.3333) -> (-25.5, -38.8333)
  line L426 (-25.5, -38.8333) -> (-27, -38.8333)
  line L427 (-27, -38.8333) -> (-27, -37.3333)
  line L428 (-25, -35) -> (-23.5, -35)
  line L429 (-23.5, -35) -> (-23.5, -36.5)
  line L430 (-23.5, -36.5) -> (-25, -36.5)
  line L431 (-25, -36.5) -> (-25, -35)
  line L432 (-27, -35) -> (-25.5, -35)
  line L433 (-25.5, -35) -> (-25.5, -36.5)
  line L434 (-25.5, -36.5) -> (-27, -36.5)
  line L435 (-27, -36.5) -> (-27, -35)
  dimension "d72" = 20.5
  dimension "d73" = 5
  dimension "d76" = -2.3
  dimension "d77" = 17
  dimension "d80" = -2.3
  dimension "d81" = 17
  dimension "d84" = -2
  dimension "d85" = 21
  dimension "d88" = -2
  dimension "d89" = 21
  dimension "d92" = -2
  dimension "d93" = 16
  dimension "d96" = -2
  dimension "d97" = 21
  constraint horizontal L4
  constraint vertical L5
  constraint horizontal L6
  constraint vertical L7
  measures "d72" distance of L0.start L0.end
  measures "d73" distance of L0.start L2.end
extrude "Extrude7" cut sketch "Sketch4" against normal blind 7 contours L4 L5 L6 L7 | L8 L9 L10 L11 | L12 L13 L14 L15 | L16 L17 L18 L19 | L20 L21 L22 L23 | L24 L25 L26 L27 | L28 L29 L30 L31 | L32 L33 L34 L35 | L36 L37 L38 L39 | L40 L41 L42 L43 | L44 L45 L46 L47 | L48 L49 L50 L51 | L52 L53 L54 L55 | L56 L57 L58 L59 | L60 L61 L62 L63 | L64 L65 L66 L67 | L68 L69 L70 L71 | L72 L73 L74 L75 | L76 L77 L78 L79 | L80 L81 L82 L83 | L84 L85 L86 L87 | L88 L89 L90 L91 | L92 L93 L94 L95 | L96 L97 L98 L99 | L100 L101 L102 L103 | L104 L105 L106 L107 | L108 L109 L110 L111 | L112 L113 L114 L115 | L116 L117 L118 L119 | L120 L121 L122 L123 | L124 L125 L126 L127 | L128 L129 L130 L131 | L132 L133 L134 L135 | L136 L137 L138 L139 | L140 L141 L142 L143 | L144 L145 L146 L147 | L148 L149 L150 L151 | L152 L153 L154 L155 | L156 L157 L158 L159 | L160 L161 L162 L163 | L164 L165 L166 L167 | L168 L169 L170 L171 | L172 L173 L174 L175 | L176 L177 L178 L179 | L180 L181 L182 L183 | L184 L185 L186 L187 | L188 L189 L190 L191 | L192 L193 L194 L195 | L196 L197 L198 L199 | L200 L201 L202 L203 | L204 L205 L206 L207 | L208 L209 L210 L211 | L212 L213 L214 L215 | L216 L217 L218 L219 | L220 L221 L222 L223 | L224 L225 L226 L227 | L228 L229 L230 L231 | L232 L233 L234 L235 | L236 L237 L238 L239 | L240 L241 L242 L243 | L244 L245 L246 L247 | L248 L249 L250 L251 | L252 L253 L254 L255 | L256 L257 L258 L259 | L260 L261 L262 L263 | L264 L265 L266 L267 | L268 L269 L270 L271 | L272 L273 L274 L275 | L276 L277 L278 L279 | L280 L281 L282 L283 | L284 L285 L286 L287 | L288 L289 L290 L291 | L292 L293 L294 L295 | L296 L297 L298 L299 | L300 L301 L302 L303 | L304 L305 L306 L307 | L308 L309 L310 L311 | L312 L313 L314 L315 | L316 L317 L318 L319 | L320 L321 L322 L323 | L324 L325 L326 L327 | L328 L329 L330 L331 | L332 L333 L334 L335 | L336 L337 L338 L339 | L340 L341 L342 L343 | L344 L345 L346 L347 | L348 L349 L350 L351 | L352 L353 L354 L355 | L356 L357 L358 L359 | L360 L361 L362 L363 | L364 L365 L366 L367 | L368 L369 L370 L371 | L372 L373 L374 L375 | L376 L377 L378 L379 | L380 L381 L382 L383 | L384 L385 L386 L387 | L388 L389 L390 L391 | L392 L393 L394 L395 | L396 L397 L398 L399 | L400 L401 L402 L403 | L404 L405 L406 L407 | L408 L409 L410 L411 | L412 L413 L414 L415 | L416 L417 L418 L419 | L420 L421 L422 L423 | L424 L425 L426 L427 | L428 L429 L430 L431 | L432 L433 L434 L435 bodies 1